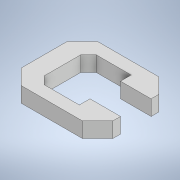
# Autodesk Inventor part: C-Clip
Saved by Autodesk Inventor 2022.2 (Build 262287030, 287C)
## iProperties
Created: 2023-03-13
Part Number: C-Clip
Material: Generic
Document SubType Name: Modeling
Designer: jak27277
Density: 1 g/cm^3
Appearance: Default
Author: jak27277
Autodesk Inventor part; units mm, degrees
ref_plane "YZ Plane" through (0, 0, 0) normal (1, 0, 0) x (0, 1, 0)
ref_plane "XZ Plane" through (0, 0, 0) normal (0, 1, 0) x (-1, 0, 0)
ref_plane "XY Plane" through (0, 0, 0) normal (0, 0, 1) x (1, 0, 0)
sketch "Sketch1" plane through (0, 0, 0) normal (0, 1, 0) x (-1, 0, 0)
  line L0 (0, 0) -> (6.35, -6.35)
  line L1 (6.35, -6.35) -> (6.35, -25.4)
  line L2 (6.35, -25.4) -> (0, -31.75)
  line L3 (0, -31.75) -> (-25.4, -31.75)
  line L4 (-25.4, -31.75) -> (-31.75, -25.4)
  line L5 (-31.75, -25.4) -> (-31.75, -22.225)
  line L6 (-31.75, -22.225) -> (-19.05, -22.225)
  line L7 (-19.05, -22.225) -> (-19.05, -26.67)
  line L8 (-19.05, -26.67) -> (-4.445, -26.67)
  line L9 (-4.445, -26.67) -> (-1.27, -23.495)
  line L10 (-1.27, -23.495) -> (-1.27, -8.255)
  line L11 (-1.27, -8.255) -> (-4.445, -5.08)
  line L12 (-4.445, -5.08) -> (-19.05, -5.08)
  line L13 (-19.05, -5.08) -> (-19.05, -9.525)
  line L14 (-19.05, -9.525) -> (-31.75, -9.525)
  line L15 (-31.75, -9.525) -> (-31.75, -6.35)
  line L16 (-31.75, -6.35) -> (-25.4, 0)
  line L17 (-25.4, 0) -> (0, 0)
  dimension "d0" = 45
  dimension "d1" = 38.1
  dimension "d2" = 31.75
  dimension "d3" = 9.525
  dimension "d4" = 5.08
  dimension "d5" = 12.7
  dimension "d6" = 5.08
  dimension "d7" = 3.175
  dimension "d8" = 7.62
  dimension "d9" = 6.35
  dimension "d10" = 31.75
  dimension "d11" = 12.7
  constraints: 36 end point, 8 perpendicular, 5 parallel, 4 point on line, 3 equal length, 2 vertical
  measures "d0" angle of L17 L16
  measures "d1" distance between parallel lines of L1 L15
  measures "d2" horizontal distance of L0.end L16.end
  measures "d3" distance between parallel lines of L17 L14
  measures "d4" distance between parallel lines of L17 L12
  measures "d5" distance of L13.end L14.end
  measures "d6" distance between parallel lines of L3 L8
  measures "d7" horizontal distance of L8.end L9.end
  measures "d8" distance between parallel lines of L1 L10
  measures "d9" horizontal distance of L1.end L2.end
  measures "d10" distance between parallel lines of L17 L3
  measures "d11" distance between parallel lines of L14 L6
extrude "Extrusion1" add sketch "Sketch1" along normal blind 6.35
body "Solid1"
